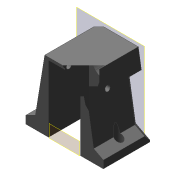
# Autodesk Inventor part: servo_clamp
Saved by Autodesk Inventor 2014 (Build 180170000, 170)
## iProperties
Created: 2015-05-30
Part Number: servo_clamp
Material: Generic
Document SubType Name: Modeling
Designer: Martin
Density: 1 g/cm^3
Appearance: Default
Author: Martin
Autodesk Inventor part; units mm, degrees
note: some values were not read from the file. Chosen so that the rebuilt part matches the saved one: sketch regions of "ext_backhousing".
ref_plane "YZ Plane" through (0, 0, 0) normal (1, 0, 0) x (0, 1, 0)
ref_plane "XZ Plane" through (0, 0, 0) normal (0, 1, 0) x (-1, 0, 0)
ref_plane "XY Plane" through (0, 0, 0) normal (0, 0, 1) x (1, 0, 0)
ref_plane "Work Plane1" through (14.3392, -46.1241, 0) normal (0, -1, 0) x (-1, 0, 0)
sketch "Sketch1" plane through (14.3392, -46.1241, 0) normal (0, -1, 0) x (-1, 0, 0)
  line L0 (-22.1702, 0) -> (47.1015, 0) projected
  line L1 (0.3, -25.8) -> (-11.3, -25.8) construction
  line L2 (-5.5, -25.8) -> (-5.5, 0) construction
  line L3 (0.8, 0) -> (0.8, -26.3)
  line L4 (0.8, -26.3) -> (-11.8, -26.3)
  line L5 (-11.8, -26.3) -> (-11.8, 0)
  line L6 (6.8, 0) -> (2.3, -27.3)
  line L7 (2.3, -27.3) -> (-13.3, -27.3)
  line L8 (-13.3, -27.3) -> (-17.8, 0)
  line L9 (5.9758, -5) -> (9.8, -3)
  line L10 (9.8, -3) -> (9.8, 0)
  line L11 (-16.9758, -5) -> (-20.8, -3)
  line L12 (-20.8, -3) -> (-20.8, 0)
  line L13 (5.9758, -5) -> (-16.9758, -5) construction
  line L14 (9.8, -3) -> (-20.8, -3) construction
  point P0 (14.3392, 0)
  dimension "d0" = 1
  dimension "d1" = 0.5
  dimension "d2" = 0.5
  dimension "d3" = 1.5
  dimension "d4" = 6
  dimension "d24" = 3
  dimension "d25" = 2
  dimension "d26" = 3
  dimension "d27" = 3
  constraints: 28 end point, 4 perpendicular, 4 vertical, 3 symmetric about line, 2 point on line, 1 horizontal, 1 midpoint, 1 parallel, 11 other
  measures "d0" distance between parallel lines of L7 L4
  measures "d1" distance from line of L5 L1.end
  measures "d2" distance from line of L1.end L4
  measures "d3" horizontal distance of L6.end L3.end
  measures "d4" distance of L3.start L6.start
  measures "d24" distance of L6.start L10.end
  measures "d25" distance between parallel lines of L14 L13
  measures "d26" distance of L9.end L10.end
  measures "d27" distance of L8.end L12.end
extrude "ext_maincage" add sketch "Sketch1" against normal blind 16 contours L0 L8 L11 L12 | L0 L5 L4 L3 L6 L7 L8 | L0 L10 L9 L6
sketch "Sketch2" plane through (14.3392, -30.1241, 0) normal (0, 1, 0) x (1, 0, 0)
  line L0 (-0.8, -26.3) -> (-0.8, 0) projected
  line L1 (-2.3, -27.3) -> (13.3, -27.3) projected
  line L2 (11.8, 0) -> (11.8, -26.3) projected
  line L3 (11.8, -26.3) -> (-0.8, -26.3) projected
  circle A0 centre (5.5, -20) radius 5.5
  circle A1 centre (5.5, -20) radius 7.3
  line L4 (-0.8, 0) -> (-0.8, -16.3122)
  line L5 (-0.8, -23.6878) -> (-0.8, -26.3)
  line L6 (-0.8, -26.3) -> (1.8122, -26.3)
  line L7 (9.1878, -26.3) -> (11.8, -26.3)
  line L8 (11.8, -23.6878) -> (11.8, -26.3)
  line L9 (-0.8, 0) -> (11.8, 0)
  line L10 (11.8, 0) -> (11.8, -16.3122)
  line L11 (-0.8, -16.3122) -> (-0.8, 0)
  line L12 (-0.8, 0) -> (-9.8, 0) projected
  line L13 (-9.8, 0) -> (-9.8, -3) projected
  line L14 (-9.8, -3) -> (-5.9758, -5) projected
  line L15 (-5.9758, -5) -> (-2.3, -27.3) projected
  line L16 (-2.3, -27.3) -> (13.3, -27.3) projected
  line L17 (13.3, -27.3) -> (16.9758, -5) projected
  line L18 (16.9758, -5) -> (20.8, -3) projected
  line L19 (20.8, -3) -> (20.8, 0) projected
  line L20 (20.8, 0) -> (11.8, 0) projected
  line L21 (11.8, 0) -> (11.8, -26.3) projected
  line L22 (11.8, -26.3) -> (-0.8, -26.3) projected
  line L23 (-0.8, -26.3) -> (-0.8, 0) projected
  point P0 (-6.8, 0)
  point P1 (17.8, 0)
  point P2 (-14.3392, 0)
  point P3 (3.5163, -12.9747)
  dimension "d7" = 11
  constraints: 16 end point, 5 point on line, 3 perpendicular, 2 coincident, 2 collinear, 1 centre point, 1 horizontal, 1 parallel, 10 other
  measures "d7" diameter of A0
extrude "ext_backhousing" add sketch "Sketch2" along normal blind 4.3
sketch "Sketch3" plane through (14.3392, -25.8241, 0) normal (0, 1, 0) x (1, 0, 0)
  line L0 (17.8, 0) -> (-6.8, 0) projected
  line L1 (-6.8, 0) -> (-2.3, -27.3) projected
  line L2 (-2.3, -27.3) -> (13.3, -27.3) projected
  line L3 (13.3, -27.3) -> (17.8, 0) projected
  circle A0 centre (5.5, -20) radius 2.5
  circle A1 centre (5.5, -20) radius 5.5 projected
  line L4 (20.8, 0) -> (-9.8, 0) projected
  line L5 (-9.8, 0) -> (-9.8, -3) projected
  line L6 (-9.8, -3) -> (-5.9758, -5) projected
  line L7 (-5.9758, -5) -> (-2.3, -27.3) projected
  line L8 (-2.3, -27.3) -> (13.3, -27.3) projected
  line L9 (13.3, -27.3) -> (16.9758, -5) projected
  line L10 (16.9758, -5) -> (20.8, -3) projected
  line L11 (20.8, -3) -> (20.8, 0) projected
  point P0 (-0.8, 0)
  point P1 (-14.3392, 0)
  dimension "d10" = 5
  constraints: 1 centre point
  measures "d10" diameter of A0
extrude "ext_backcover" add sketch "Sketch3" along normal blind 1 contours L3 L2 L1 L0 | L4 L11 L10 L3 | L1 L6 L5 L4 | A1
sketch "Sketch4" plane through (14.3392, -24.8241, 0) normal (0, 1, 0) x (1, 0, 0)
  circle A0 centre (5.5, -20) radius 2.5 projected
  line L0 (5.5, 0) -> (5.5, -17.5)
  line L1 (5.5, -15) -> (2.6132, -10)
  line L2 (2.6132, -10) -> (2.6132, 0)
  line L3 (20.8, 0) -> (-9.8, 0) projected
  line L4 (13.3, -27.3) -> (16.9758, -5) projected
  line L5 (20.8, -3) -> (20.8, 0) projected
  line L6 (8, -20) -> (14.5033, -20)
  line L7 (-2.3, -27.3) -> (13.3, -27.3) projected
  line L8 (16.9758, -5) -> (20.8, -3) projected
  circle A1 centre (5.5, -20) radius 2.5
  line L9 (14.5643, -19.6299) -> (16.9758, -5)
  line L10 (16.9758, -5) -> (20.8, -3)
  line L11 (20.8, -3) -> (20.8, 0)
  line L12 (20.8, 0) -> (5.5, 0)
  point P0 (-14.3392, 0)
  dimension "d22" = 30
  dimension "d23" = 10
  dimension "d28" = 5
  constraints: 16 end point, 4 point on line, 3 collinear, 2 line through centre, 2 perpendicular, 2 point on circle, 1 centre point, 1 coincident, 1 concentric, 1 midpoint, 1 parallel
  measures "d22" angle of L0 L1
  measures "d23" distance of L1.end L2.end
  measures "d28" vertical distance of L1.end L1.start
extrude "ext_cut_backcutway" cut sketch "Sketch4" against normal blind 3 contours A0 L0 L3 L5 L8 L4 L6 | L1 L2 L3 L0
chamfer "Chamfer3" distance 2 angle 45 4 edges at (30.0788, -27.8241, 12.5) (33.2272, -27.8241, 4) (6.4513, -24.8241, 4) (10.2013, -24.8241, 16.15)
ref_plane "back_plane" through (14.3392, -24.8241, 0) normal (0, 1, 0) x (1, 0, 0)
sketch "Sketch5" plane through (14.3392, -24.8241, 0) normal (0, 1, 0) x (1, 0, 0)
  line L0 (-0.273, -27.3) -> (13.3, -27.3) projected
  line L1 (2.6132, 0) -> (20.8, 0) projected
  line L2 (11, -9) -> (11, -3)
  line L3 (11, -3) -> (0, -3)
  line L4 (0, -3) -> (0, -9)
  line L5 (0, -9) -> (11, -9)
  line L6 (11, -9) -> (0, -3) construction
  line L7 (11, -3) -> (0, -9) construction
  arc A0 (5.5, -17.5) -> (8, -20) centre (5.5, -20) ccw projected
  line L8 (5.5, -20) -> (5.5, -3) construction
  point P0 (-14.3392, 0)
  point P1 (5.5, -6)
  point P2 (5.5, -6)
  dimension "d33" = 6
  dimension "d34" = 11
  dimension "d37" = 3
  constraints: 14 end point, 4 midpoint, 3 parallel, 2 perpendicular, 1 coincident, 1 point on line
  measures "d33" distance of L2.start L2.end
  measures "d34" distance of L4.end L2.start
  measures "d37" distance between parallel lines of L1 L3
extrude "Extrusion5" cut sketch "Sketch5" against normal through all
sketch "Sketch6" plane through (0, 0, 0) normal (0, 0, 1) x (1, 0, 0)
  line L0 (35.1392, -46.1241) -> (35.1392, -27.8241) projected
  circle A0 centre (32.1392, -36.9741) radius 1.5
  line L1 (33.6392, -36.9741) -> (35.1392, -36.9741)
  line L2 (32.1392, -36.9741) -> (33.6392, -36.9741) construction
  line L3 (4.5392, -46.1241) -> (4.5392, -26.8241) projected
  line L4 (4.5392, -46.1241) -> (4.5392, -24.8241) projected
  circle A1 centre (7.5392, -31.1241) radius 1.5
  circle A2 centre (7.5392, -41.1241) radius 1.5
  line L5 (7.5392, -31.1241) -> (7.5392, -41.1241) construction
  line L6 (7.5392, -41.1241) -> (6.0392, -41.1241) construction
  line L7 (7.5392, -31.1241) -> (6.0392, -31.1241) construction
  line L8 (4.5392, -31.1241) -> (6.0392, -31.1241)
  line L9 (4.5392, -41.1241) -> (6.0392, -41.1241)
  line L10 (35.1392, -46.1241) -> (35.1392, -29.8241) projected
  point P0 (0, 0)
  dimension "d38" = 3
  dimension "d40" = 1.5
  dimension "d43" = 10
  dimension "d44" = 5
  constraints: 14 end point, 3 perpendicular, 2 equal length, 2 horizontal alignment, 2 parallel, 2 point on circle, 2 point on line, 1 centre point, 1 collinear, 1 midpoint, 5 other
  measures "d40" distance of L1.start L1.end
  measures "d43" distance of L5.start L5.end
  measures "d44" distance from line of L9 L3.start
extrude "Extrusion6" cut sketch "Sketch6" along normal through all
sketch "Sketch7" plane through (26.1392, -46.1241, 0) normal (-1, 0, 0) x (0, 0, 1)
  line L0 (26.3, 0) -> (26.3, 16) projected
  line L1 (0, 0) -> (0, 16) projected
  line L2 (26.3, 8) -> (0, 8) construction
  circle A0 centre (20.3, 8) radius 1
  point P0 (0, 46.1241)
  dimension "d47" = 2
  dimension "d48" = 6
  constraints: 2 end point, 2 midpoint, 1 centre point, 1 point on line
  measures "d47" diameter of A0
  measures "d48" distance from line of L0 A0.centre
extrude "Extrusion7" cut sketch "Sketch7" along normal through all both and the other way through all
equation "\"d7\" = linact_bearing_diameter"
equation "\"d8\" = linact_bearing_thickness"
equation "\"d38\" = screw_m3_bore_selfthreading"
equation "\"d47\" = screw_m2_bore_selfthreading"
equation "\"linact_bearing_diameter\" = 11"
equation "\"linact_bearing_thickness\" = 4.3"
equation "\"screw_m3_bore_selfthreading\" = 3"
equation "\"screw_m2_bore_selfthreading\" = 2"
body "Solid1"
